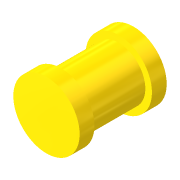
# Autodesk Inventor part: 00_Threaded_Insert_M3_8mm
Saved by Autodesk Inventor 2022 (Build 260153000, 153)
## iProperties
Created: 2021-12-20
Part Number: 00_Threaded_Insert_M3_8mm
Material: Generisch
Document SubType Name: Modeling
Designer: diederichbenedict
Density: 1 g/cm^3
Appearance: Glänzend - Gold
Author: diederichbenedict
Autodesk Inventor part; units mm, degrees
ref_plane "YZ Plane" through (0, 0, 0) normal (1, 0, 0) x (0, 1, 0)
ref_plane "XZ Plane" through (0, 0, 0) normal (0, 1, 0) x (-1, 0, 0)
ref_plane "XY Plane" through (0, 0, 0) normal (0, 0, 1) x (1, 0, 0)
sketch "Skizze1" plane through (0, 0, 0) normal (1, 0, 0) x (0, 1, 0)
  line L0 (0, 0) -> (2.25, 0)
  line L1 (2.25, 0) -> (2.25, 1)
  line L2 (2.25, 1) -> (1.8, 1)
  line L3 (1.8, 1) -> (1.8, 4.9)
  line L4 (1.8, 4.9) -> (2.25, 4.9)
  line L5 (2.25, 4.9) -> (2.25, 5.9)
  line L6 (2.25, 5.9) -> (0, 5.9)
  line L7 (0, 5.9) -> (0, 0)
  dimension "d0" = 2.25
  dimension "d1" = 1
  dimension "d3" = 3.9
  dimension "d4" = 1
  dimension "d5" = 1.8
  constraints: 16 end point, 6 perpendicular, 2 point on line, 1 horizontal
  measures "d0" distance of L0.start L0.end
  measures "d1" distance of L0.end L1.end
  measures "d3" distance of L2.end L3.end
  measures "d4" distance of L4.end L5.end
  measures "d5" distance between parallel lines of L3 L7
revolve "Umdrehung1" add sketch "Skizze1" angle 360 about axis through (0, 0, 5.9) along (0, 0, -1)
